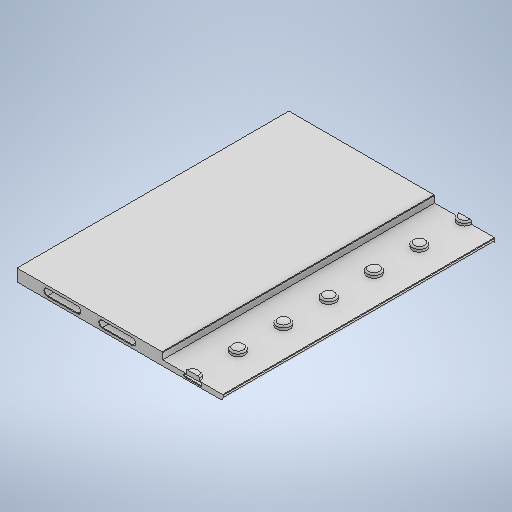
# Autodesk Inventor part: RightFlap5
Saved by Autodesk Inventor 2025.3 (Build 293356000, 356)
## iProperties
Created: 2025-11-19
Part Number: RightFlap5
Material: Generic
Document SubType Name: Modeling
Designer: User
Density: 1 g/cm^3
Appearance: Default
Author: User
Autodesk Inventor part; units mm, degrees
ref_plane "YZ Plane" through (0, 0, 0) normal (1, 0, 0) x (0, 1, 0)
ref_plane "XZ Plane" through (0, 0, 0) normal (0, 1, 0) x (-1, 0, 0)
ref_plane "XY Plane" through (0, 0, 0) normal (0, 0, 1) x (1, 0, 0)
sketch "Sketch1" plane through (0, 0, 0) normal (0, 1, 0) x (-1, 0, 0)
  line L0 (0, 0) -> (300, 0)
  line L1 (300, 0) -> (300, -420)
  line L2 (300, -420) -> (0, -420)
  line L3 (0, -420) -> (0, 0)
  line L4 (240, -150) -> (280, -150)
  line L5 (280, -150) -> (280, -270)
  line L6 (280, -270) -> (240, -270)
  line L7 (240, -270) -> (240, -150)
  line L8 (240, -150) -> (280, -270) construction
  line L9 (280, -150) -> (240, -270) construction
  dimension "d0" = 300
  dimension "d1" = 420
  dimension "d5" = 40
  dimension "d6" = 120
  constraints: 20 end point, 4 parallel, 2 horizontal, 2 perpendicular
  measures "d0" distance of L1.end L2.end
  measures "d1" distance of L0.end L1.end
  measures "d5" distance of L5.end L6.end
  measures "d6" distance of L4.end L5.end
extrude "Extrusion1" add sketch "Sketch1" along normal blind 8
sketch "Sketch2" plane through (0, 0, 0) normal (1, 0, 0) x (0, 0, -1)
  line L0 (150, 0) -> (270, 0) projected
  line L1 (210, 0) -> (210, 4)
  line L2 (420, 0) -> (420, 8) projected
  line L3 (0, 4.5) -> (420, 4.5)
  line L4 (420, 4.5) -> (420, 3.5)
  line L5 (420, 3.5) -> (0, 3.5)
  line L6 (0, 3.5) -> (0, 4.5)
  line L7 (0, 4.5) -> (420, 3.5) construction
  line L8 (420, 4.5) -> (0, 3.5) construction
  line L9 (0, 0) -> (0, 8) projected
  line L10 (420, 3.5) -> (0, 3.5)
  line L11 (0, 3.5) -> (0, 8)
  line L12 (0, 8) -> (420, 8)
  line L13 (420, 8) -> (420, 3.5)
  dimension "d7" = 4
  dimension "d8" = 1
  constraints: 22 end point, 4 parallel, 3 midpoint, 2 horizontal, 2 perpendicular, 1 point on line, 1 vertical
  measures "d7" distance of L1.start L1.end
  measures "d8" distance of L3.end L4.end
extrude "Extrusion2" cut sketch "Sketch2" against normal blind 40
fillet "Fillet1" radius 3.1 14 edges at (-300, 8, -210) (-300, 0, -210) (-280, 8, -210) (-260, 8, -270) (-240, 8, -210) (-280, 0, -210) (-260, 0, -270) (-280, 4, -270) (-240, 4, -270) (-240, 4, -150) (-260, 0, -150) (-260, 8, -150) (-280, 4, -150) (-240, 0, -210)
fillet "Fillet2" radius 2 11 edges at (-299.092, 7.092, 0) (-300, 4, 0) (-299.092, 0.908, 0) (-148.45, 0, 0) (-168.45, 8, 0) (-299.092, 7.092, -420) (-300, 4, -420) (-299.092, 0.908, -420) (-148.45, 0, -420) (-168.45, 8, -420) (0, 0, -210)
fillet "Fillet3" radius 0.3 8 edges at (-40, 7.4142, -419.4142) (-40, 4.75, -420) (-40, 7.4142, -0.5858) (-40, 4.75, 0) (-40, 8, -210) (-20, 3.5, -420) (0, 3.5, -210) (-20, 3.5, 0)
fillet "Fillet4" radius 2 6 edges at (-0.0879, 3.4121, -0.0879) (-0.5858, 0.5858, -0.5858) (0, 2.6, 0) (-0.0879, 3.4121, -419.9121) (-0.5858, 0.5858, -419.4142) (0, 2.6, -420)
mirror "Mirror1" about plane through (0, 0, 0) normal (1, 0, 0) remove original yes
sketch "Sketch3" plane through (2, 3.5, -0.3) normal (0, 1, 0) x (1, 0, 0)
  circle A0 centre (18, 14.7) radius 4.5
  line L0 (-1.7, 417.7) -> (-1.7, 1.7) construction
  line L1 (0, 0) -> (38, 0) projected
  circle A1 centre (18, 44.7) radius 4.5
  circle A2 centre (18, 74.7) radius 4.5
  line L2 (-2, 1.7) -> (-2, 417.7) projected
  line L3 (18, 74.7) -> (5.7787, 74.7)
  circle A3 centre (18, 134.7) radius 4.5
  circle A4 centre (18, 104.7) radius 4.5
  circle A5 centre (18, 74.7) radius 4.5
  line L4 (18, 134.7) -> (3.7207, 134.7)
  circle A6 centre (18, 194.7) radius 4.5
  line L5 (18, 194.7) -> (5.7787, 194.7)
  circle A7 centre (18, 164.7) radius 4.5
  circle A8 centre (18, 134.7) radius 4.5
  circle A9 centre (18, 254.7) radius 4.5
  line L6 (18, 254.7) -> (3.7207, 254.7)
  circle A10 centre (18, 224.7) radius 4.5
  circle A11 centre (18, 374.7) radius 4.5
  circle A12 centre (18, 344.7) radius 4.5
  circle A13 centre (18, 314.7) radius 4.5
  line L7 (18, 314.7) -> (5.7787, 314.7)
  circle A14 centre (18, 314.7) radius 4.5
  circle A15 centre (18, 284.7) radius 4.5
  circle A16 centre (18, 254.7) radius 4.5
  line L8 (18, 254.7) -> (3.7207, 254.7)
  circle A17 centre (18, 254.7) radius 4.5
  circle A18 centre (18, 224.7) radius 4.5
  circle A19 centre (18, 404.7) radius 4.5
  line L9 (0, 419.7) -> (38.3, 419.7) projected
  line L10 (38.3, -0.3) -> (0, -0.3) projected
  point P0 (-2, -0.3)
  dimension "d15" = 9
  dimension "d18" = 9
  dimension "d19" = 9
  dimension "d20" = 30
  dimension "d21" = 30
  dimension "d23" = 20
  dimension "d24" = 20
  dimension "d25" = 30
  dimension "d26" = 15
  dimension "d27" = 15
  constraints: 20 centre point, 14 symmetric about line, 12 end point, 2 horizontal, 16 other
  measures "d15" diameter of A0
  measures "d18" diameter of A1
  measures "d19" diameter of A2
  measures "d20" distance of A1.centre A0.centre
  measures "d21" distance of A1.centre L3.start
  measures "d23" distance from line of L2 A0.centre
  measures "d24" distance from line of L2 A19.centre
  measures "d25" distance of A19.centre A11.centre
  measures "d26" distance from line of L9 A19.centre
  measures "d27" distance from line of L10 A0.centre
extrude "Extrusion3" add sketch "Sketch3" along normal blind 2.5
fillet "Fillet5" radius 1 14 edges at (15.5, 6, -15) (15.5, 6, -45) (15.5, 6, -75) (15.5, 6, -105) (15.5, 6, -135) (15.5, 6, -165) (15.5, 6, -195) (15.5, 6, -225) (15.5, 6, -255) (15.5, 6, -285) (15.5, 6, -315) (15.5, 6, -345) (15.5, 6, -375) (15.5, 6, -405)
sketch "Sketch4" plane through (40.3, 8, -2) normal (0, 1, 0) x (1, 0, 0)
  line L0 (276.109, -16.9477) -> (96.109, -16.9477)
  line L1 (96.109, -16.9477) -> (96.109, 163.0523)
  line L2 (96.109, 163.0523) -> (276.109, 163.0523)
  line L3 (276.109, 163.0523) -> (276.109, -16.9477)
  line L4 (276.109, 163.0523) -> (96.109, 163.0523)
  line L5 (96.109, 163.0523) -> (96.109, 343.0523)
  line L6 (96.109, 343.0523) -> (276.109, 343.0523)
  line L7 (276.109, 343.0523) -> (276.109, 163.0523)
  line L8 (276.109, 343.0523) -> (96.109, 343.0523)
  line L9 (96.109, 343.0523) -> (96.109, 523.0523)
  line L10 (96.109, 523.0523) -> (276.109, 523.0523)
  line L11 (276.109, 523.0523) -> (276.109, 343.0523)
  line L12 (96.109, 163.0523) -> (-83.891, 163.0523)
  line L13 (-83.891, 163.0523) -> (-83.891, -16.9477)
  line L14 (-83.891, -16.9477) -> (96.109, -16.9477)
  line L15 (96.109, -16.9477) -> (96.109, 163.0523)
  line L16 (96.109, 163.0523) -> (-83.891, 163.0523)
  line L17 (-83.891, 163.0523) -> (-83.891, 343.0523)
  line L18 (-83.891, 343.0523) -> (96.109, 343.0523)
  line L19 (96.109, 343.0523) -> (96.109, 163.0523)
  line L20 (96.109, 343.0523) -> (-83.891, 343.0523)
  line L21 (-83.891, 343.0523) -> (-83.891, 523.0523)
  line L22 (-83.891, 523.0523) -> (96.109, 523.0523)
  line L23 (96.109, 523.0523) -> (96.109, 343.0523)
  point P0 (-40.3, -2)
  dimension "d31" = 180
  dimension "d32" = 180
  dimension "d33" = 180
  dimension "d34" = 180
  dimension "d35" = 180
  constraints: 48 end point, 12 parallel, 6 horizontal, 6 perpendicular, 5 point on line
  measures "d31" distance of L1.end L2.end
  measures "d32" distance of L0.end L1.end
  measures "d33" distance of L4.end L5.end
  measures "d34" distance of L8.end L9.end
  measures "d35" distance of L14.end L13.end
extrude "Extrusion4" cut sketch "Sketch4" against normal through all contours L0 L1 L2 L3 | L14 L13 L12 L1 | L2 L5 L6 L7 | L6 L9 L10 L11 | L18 L21 L22 L9
sketch "Sketch5" plane through (40.3, 8, -165.0523) normal (0, 0, 1) x (1, 0, 0)
  line L0 (-15.3, -6) -> (-25.3, -6) construction
  line L1 (-40.3, -6) -> (-40.3, -4.8) projected
  line L2 (-15.3, -5.25) -> (-25.3, -5.25)
  line L3 (-25.3, -6.75) -> (-15.3, -6.75)
  arc A0 (-15.3, -6.75) -> (-15.3, -5.25) centre (-15.3, -6) ccw
  arc A1 (-25.3, -5.25) -> (-25.3, -6.75) centre (-25.3, -6) ccw
  line L4 (76.109, -4) -> (56.109, -4) construction
  line L5 (96.109, 0) -> (96.109, -8) projected
  line L6 (76.109, -2) -> (56.109, -2)
  line L7 (56.109, -6) -> (76.109, -6)
  arc A2 (76.109, -6) -> (76.109, -2) centre (76.109, -4) ccw
  arc A3 (56.109, -2) -> (56.109, -6) centre (56.109, -4) ccw
  line L8 (39.7, -4) -> (19.7, -4) construction
  line L9 (39.7, -2) -> (19.7, -2)
  line L10 (19.7, -6) -> (39.7, -6)
  arc A4 (39.7, -6) -> (39.7, -2) centre (39.7, -4) ccw
  arc A5 (19.7, -2) -> (19.7, -6) centre (19.7, -4) ccw
  line L11 (29.7, -4) -> (49.7, -4) construction
  line L12 (-0.3, -4.5) -> (-0.3, -0.3) projected
  point P0 (-40.3, -8)
  point P1 (-20.3, -6)
  point P2 (66.109, -4)
  dimension "d48" = 5
  dimension "d49" = 1.5
  dimension "d50" = 20
  dimension "d51" = 10
  dimension "d52" = 4
  dimension "d53" = 30
  dimension "d54" = 10
  dimension "d55" = 180
  dimension "d56" = 4
  dimension "d57" = 30
  constraints: 26 end point, 12 point on circle, 12 tangent, 6 centre point, 3 midpoint, 3 parallel, 2 horizontal, 2 perpendicular, 1 collinear
  measures "d48" distance of point (-20.3, -6) L0.end
  measures "d49" diameter of A1
  measures "d50" distance from line of L1 point (-20.3, -6)
  measures "d51" distance of point (66.109, -4) L4.end
  measures "d52" diameter of A3
  measures "d53" distance from line of L5 point (66.109, -4)
  measures "d54" distance of L11.start L8.end
  measures "d55" angle of L8 L11
  measures "d56" diameter of A5
  measures "d57" distance from line of L12 L11.start
extrude "Extrusion5" cut sketch "Sketch5" against normal blind 16
sketch "Sketch6" plane through (136.409, 8, -345.0523) normal (0, 0, -1) x (-1, 0, 0)
  line L0 (111.409, -6) -> (121.409, -6) construction
  line L1 (111.409, -6.75) -> (121.409, -6.75)
  line L2 (121.409, -5.25) -> (111.409, -5.25)
  arc A0 (111.409, -5.25) -> (111.409, -6.75) centre (111.409, -6) ccw
  arc A1 (121.409, -6.75) -> (121.409, -5.25) centre (121.409, -6) ccw
  line L3 (136.409, -4.8) -> (136.409, -6) projected
  line L4 (20, -4) -> (40, -4) construction
  line L5 (20, -6) -> (40, -6)
  line L6 (40, -2) -> (20, -2)
  arc A2 (20, -2) -> (20, -6) centre (20, -4) ccw
  arc A3 (40, -6) -> (40, -2) centre (40, -4) ccw
  line L7 (0, 0) -> (0, -8) projected
  line L8 (56.409, -4) -> (76.409, -4) construction
  line L9 (56.409, -6) -> (76.409, -6)
  line L10 (76.409, -2) -> (56.409, -2)
  arc A4 (56.409, -2) -> (56.409, -6) centre (56.409, -4) ccw
  arc A5 (76.409, -6) -> (76.409, -2) centre (76.409, -4) ccw
  line L11 (96.409, -0.3) -> (96.409, -4.5) projected
  point P0 (136.409, -8)
  point P1 (116.409, -6)
  point P2 (30, -4)
  point P3 (0, -4)
  point P4 (66.409, -4)
  dimension "d60" = 5
  dimension "d61" = 1.5
  dimension "d62" = 20
  dimension "d63" = 10
  dimension "d64" = 4
  dimension "d65" = 30
  dimension "d66" = 10
  dimension "d67" = 4
  dimension "d68" = 30
  constraints: 24 end point, 12 point on circle, 12 tangent, 6 centre point, 4 midpoint, 3 horizontal, 3 parallel
  measures "d60" distance of point (116.409, -6) L0.end
  measures "d61" diameter of A1
  measures "d62" distance from line of L3 point (116.409, -6)
  measures "d63" distance of point (30, -4) L4.end
  measures "d64" diameter of A3
  measures "d65" distance of point (0, -4) point (30, -4)
  measures "d66" distance of point (66.409, -4) L8.end
  measures "d67" diameter of A5
  measures "d68" distance from line of L11 point (66.409, -4)
extrude "Extrusion6" cut sketch "Sketch6" against normal blind 16
sketch "Sketch7" plane through (136.409, 8, -165.0523) normal (1, 0, 0) x (0, 0, -1)
  line L0 (20, -4) -> (40, -4) construction
  line L1 (20, -6) -> (40, -6)
  line L2 (40, -2) -> (20, -2)
  arc A0 (20, -2) -> (20, -6) centre (20, -4) ccw
  arc A1 (40, -6) -> (40, -2) centre (40, -4) ccw
  line L3 (0, 0) -> (0, -8) projected
  line L4 (160, -4) -> (140, -4) construction
  line L5 (0, -4.8) -> (180, -4.8) projected
  line L6 (160, -2) -> (140, -2)
  line L7 (140, -6) -> (160, -6)
  arc A2 (160, -6) -> (160, -2) centre (160, -4) ccw
  arc A3 (140, -2) -> (140, -6) centre (140, -4) ccw
  line L8 (150, -4) -> (170, -4) construction
  line L9 (180, 0) -> (180, -8) projected
  point P0 (-165.0523, -8)
  point P1 (30, -4)
  dimension "d71" = 10
  dimension "d72" = 4
  dimension "d73" = 30
  dimension "d74" = 10
  dimension "d75" = 180
  dimension "d76" = 4
  dimension "d77" = 30
  constraints: 18 end point, 8 point on circle, 8 tangent, 4 centre point, 3 parallel, 2 horizontal, 2 midpoint, 1 collinear
  measures "d71" distance of point (30, -4) L0.end
  measures "d72" diameter of A1
  measures "d73" distance from line of L3 point (30, -4)
  measures "d74" distance of L8.start L4.end
  measures "d75" angle of L4 L8
  measures "d76" diameter of A3
  measures "d77" distance from line of L9 L8.start
extrude "Extrusion7" cut sketch "Sketch7" against normal blind 16
chamfer "Chamfer1" distance 0.3 angle 45 32 edges at (136.409, 2, -195.0523) (136.409, 4, -183.0523) (136.409, 6, -195.0523) (136.409, 4, -207.0523) (106.409, 2, -165.0523) (94.409, 4, -165.0523) (106.409, 6, -165.0523) (118.409, 4, -165.0523) (82, 4, -165.0523) (70, 2, -165.0523) (58, 4, -165.0523) (70, 6, -165.0523) (25.75, 2, -165.0523) (20, 1.25, -165.0523) (14.25, 2, -165.0523) (20, 2.75, -165.0523) (136.409, 4, -327.0523) (136.409, 2, -315.0523) (136.409, 4, -303.0523) (136.409, 6, -315.0523) (118.409, 4, -345.0523) (106.409, 6, -345.0523) (94.409, 4, -345.0523) (106.409, 2, -345.0523) (82, 4, -345.0523) (70, 6, -345.0523) (58, 4, -345.0523) (70, 2, -345.0523) (20, 2.75, -345.0523) (14.25, 2, -345.0523) (20, 1.25, -345.0523) (25.75, 2, -345.0523)
mirror "Mirror2" about plane through (0, 0, 0) normal (-1, 0, 0) remove original yes
body "Solid1"
